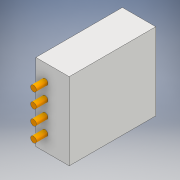
# Autodesk Inventor part: Female USB SMT
Saved by Autodesk Inventor 2018.1 (Build 221171000, 171)
## iProperties
Created: 2017-10-19
Part Number: Female USB SMT
Material: Generic
Document SubType Name: Modeling
Designer: xdlea
Density: 1 g/cm^3
Appearance: Default
Author: xdlea
Autodesk Inventor part; units mm, degrees
ref_plane "YZ Plane" through (0, 0, 0) normal (1, 0, 0) x (0, 1, 0)
ref_plane "XZ Plane" through (0, 0, 0) normal (0, 1, 0) x (-1, 0, 0)
ref_plane "XY Plane" through (0, 0, 0) normal (0, 0, 1) x (1, 0, 0)
sketch "Sketch1" plane through (0, 0, 0) normal (0, 1, 0) x (-1, 0, 0)
  line L0 (-2.875, 6.65) -> (2.875, 6.65)
  line L1 (2.875, 6.65) -> (2.875, -6.65)
  line L2 (2.875, -6.65) -> (-2.875, -6.65)
  line L3 (-2.875, -6.65) -> (-2.875, 6.65)
  line L4 (-2.875, 6.65) -> (2.875, -6.65) construction
  line L5 (2.875, 6.65) -> (-2.875, -6.65) construction
  line L6 (2.475, -6.25) -> (2.475, 6.25)
  line L7 (2.475, 6.25) -> (-2.475, 6.25)
  line L8 (-2.475, 6.25) -> (-2.475, -6.25)
  line L9 (-2.475, -6.25) -> (2.475, -6.25)
  circle A0 centre (1.285, 3.81) radius 0.5
  point P0 (0, 0)
  dimension "d0" = 13.3
  dimension "d1" = 5.75
  dimension "d2" = 0.4
  dimension "d7" = 1
  dimension "d8" = 4.16
  dimension "d9" = 3.81
  constraints: 20 end point, 4 parallel, 2 midpoint, 2 perpendicular, 1 centre point, 1 horizontal, 3 other
  measures "d0" distance of L0.end L1.end
  measures "d1" distance of L1.end L2.end
  measures "d2" distance between parallel lines of L6 L1
  measures "d7" diameter of A0
  measures "d8" distance from line of L3 A0.centre
  measures "d9" vertical distance of point (0, 0) A0.centre
extrude "Extrusion1" add sketch "Sketch1" along normal blind 14.9 contours L0 L1 L2 L3
extrude "Extrusion2" add sketch "Sketch1" along normal blind 0.4 contours L9 L8 L7 L6 | A0
extrude "Extrusion3" add sketch "Sketch1" against normal blind 2 contours A0
pattern_linear "Rectangular Pattern1" count 4 spacing 2.54 along (0, 0, -1) of "Extrusion3"
body "Solid1"
